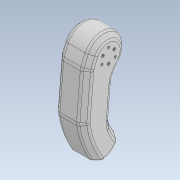
# Autodesk Inventor part: thigh_link
Saved by Autodesk Inventor 2020 (Build 240168000, 168)
## iProperties
Created: 2020-12-22
Part Number: thigh_link
Material: Generic
Document SubType Name: Modeling
Designer: DELL
Density: 1 g/cm^3
Appearance: Default
Author: DELL
Autodesk Inventor part; units mm, degrees
ref_plane "YZ Plane" through (0, 0, 0) normal (1, 0, 0) x (0, 1, 0)
ref_plane "XZ Plane" through (0, 0, 0) normal (0, 1, 0) x (-1, 0, 0)
ref_plane "XY Plane" through (0, 0, 0) normal (0, 0, 1) x (1, 0, 0)
sketch "Sketch1" plane through (0, 0, 0) normal (1, 0, 0) x (0, 1, 0)
  circle A0 centre (0, 0) radius 11.5 construction
  line L0 (0, 0) -> (-120, 0) construction
  circle A1 centre (11.5, 0) radius 1.65
  circle A2 centre (-5.75, 9.9593) radius 1.65
  circle A3 centre (-5.75, -9.9593) radius 1.65
  line L1 (0, 0) -> (-5.75, 9.9593) construction
  line L2 (0, 0) -> (-5.75, -9.9593) construction
  line L3 (0, 11.5) -> (0, -11.5) construction
  circle A4 centre (0, 0) radius 9.715 construction
  circle A5 centre (-9.715, 0) radius 2
  circle A6 centre (4.8575, 8.4134) radius 2
  circle A7 centre (4.8575, -8.4134) radius 2
  line L4 (0, 0) -> (5.75, 9.9593) construction
  line L5 (0, 0) -> (5.75, -9.9593) construction
  circle A8 centre (0, 0) radius 27.5
  circle A9 centre (-120, 0) radius 20
  circle A10 centre (11.5, 0) radius 2.75
  circle A11 centre (-5.75, 9.9593) radius 2.75
  circle A12 centre (-5.75, -9.9593) radius 2.75
  arc A13 (-75.8304, 37.2483) -> (-3.0292, 30.8791) centre (-52.1094, -110.8642) ccw
  arc A14 (-91.8203, -7.8005) -> (-28.6747, -13.325) centre (-66.1719, -78.2786) ccw
  line L6 (-7.8301, 31.9039) -> (-70.9245, 37.4239)
  line L7 (-36.9309, -10.7221) -> (-83.2376, -6.6707)
  arc A15 (-3.0292, 30.8791) -> (-7.8301, 31.9039) centre (-9.5733, 11.98) ccw
  arc A16 (-70.9245, 37.4239) -> (-75.8304, 37.2483) centre (-72.6676, 17.5) ccw
  arc A17 (-28.6747, -13.325) -> (-36.9309, -10.7221) centre (-38.674, -30.646) ccw
  arc A18 (-83.2376, -6.6707) -> (-91.8203, -7.8005) centre (-84.9807, -26.5946) ccw
  line L8 (-130.4447, 17.056) -> (-108.6678, -16.4797) construction
  arc A19 (-130.4447, 17.056) -> (-108.6678, -16.4797) centre (-106.9681, 8.4625) ccw
  point P0 (-60, 0)
  point P1 (14.3, 23.4896)
  point P2 (-14.3, -23.4896)
  point P3 (-108.2237, -16.1653)
  point P4 (-17.7534, -21.0016)
  point P5 (11.698, 24.8879)
  point P6 (-130.0481, 17.2927)
  point P7 (-5.4557, 31.6961)
  point P8 (-73.299, 37.6316)
  point P9 (-32.8704, -11.0773)
  point P10 (-87.2981, -6.3155)
  dimension "d0" = 23
  dimension "d1" = 120
  dimension "d2" = 3.3
  dimension "d3" = 30
  dimension "d4" = 30
  dimension "d5" = 19.43
  dimension "d6" = 4
  dimension "d7" = 30
  dimension "d8" = 55
  dimension "d12" = 5.5
  dimension "d25" = 40
  dimension "d26" = 150
  dimension "d27" = 300
  dimension "d28" = 20
  dimension "d29" = 45
  dimension "d30" = 5
  dimension "d35" = 25
  dimension "d36" = 17.5
  constraints: 27 point on circle, 19 centre point, 18 end point, 12 tangent, 9 equal radius, 7 coincident, 7 point on line, 3 midpoint, 2 horizontal alignment, 1 horizontal, 1 parallel, 1 vertical, 10 other
  measures "d1" distance of L0.end point (0, 0)
  measures "d2" diameter of A1
  measures "d3" angle of L3 L1
  measures "d4" angle of L3 L2
  measures "d5" diameter of A4
  measures "d6" diameter of A6
  measures "d7" angle of L3 L4
  measures "d8" diameter of A8
  measures "d12" diameter of A10
  measures "d25" diameter of A9
  measures "d26" diameter of A14
  measures "d27" diameter of A13
  measures "d28" radius of A15
  measures "d29" distance between parallel lines of L7 L6
  measures "d30" angle of L0 L6
  measures "d35" radius of A19
  measures "d36" distance from line of L0 A16.centre
extrude "Extrusion1" add sketch "Sketch1" against normal mid plane 45 contours A5 | A6 | A7 | A8 | A8 A14 A17 L7 A18 A9 A13 A16 L6 A15 | A9 A19 | A10 | A11 | A12 picked at (-121.0758, 2.6201)
extrude "Extrusion2" cut sketch "Sketch1" along normal blind 35 from surface at -22.5 contours A10 | A11 | A12
extrude "Extrusion3" cut sketch "Sketch1" against normal blind 5 from surface at 22.5 contours A5 | A6 | A7
chamfer "Chamfer1" distance 8 angle 45 1 edges at (22.5, 23.1436, -14.8534)
chamfer "Chamfer2" distance 8 angle 45 1 edges at (-22.5, 23.1436, -14.8534)
fillet "Fillet1" radius 5 12 edges at (-14.5, 23.1436, -14.8534) (-22.5, 16.4109, -10.5324) (14.5, 23.1436, -14.8534) (22.5, 16.4109, -10.5324) (22.5, -127.8077, -5.3474) (18.3996, -131.7693, 11.6088) (0, -130.4447, 17.056) (-18.3996, -131.7693, 11.6088) (-22.5, -127.8077, -5.3474) (18.3926, -113.9917, -15.5306) (0, -108.6678, -16.4797) (-18.3926, -113.9917, -15.5306)
equation "\"d1\" = shank_length"
equation "\"shank_length\" = 120"
body "Solid1"
